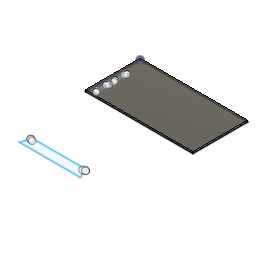
Zaagblad_E (Autodesk Fusion 360 archive; units mm, degrees)
design "Zaagblad_E" references "autodesk generic router xyz"
Autodesk Fusion 360 part; units mm, degrees
sketch "Sketch1" plane through (0, 0, 0) normal (0, 0, 1) x (1, 0, 0)
  line L0 (50.1556, -434.7837) -> (50.1556, -539.8131)
  line L1 (66.9337, -559.4908) -> (52.2058, -544.7629)
  arc A0 (50.1556, -539.8131) -> (52.2058, -544.7629) centre (57.1556, -539.8131) ccw construction
  arc A1 (51.62, -431.2482) -> (50.1556, -434.7837) centre (55.1556, -434.7837) ccw construction
  line L2 (67.2266, -415.6416) -> (51.62, -431.2482) construction
  line L3 (50.1556, -434.7837) -> (50.1556, -539.8131) construction
  line L4 (67.2266, -559.7837) -> (52.2058, -544.7629) construction
  arc A2 (50.1556, -539.8131) -> (52.2058, -544.7629) centre (57.1556, -539.8131) ccw
  arc A3 (51.62, -431.2482) -> (50.1556, -434.7837) centre (55.1556, -434.7837) ccw
  line L5 (66.9337, -415.9345) -> (51.62, -431.2482)
  line L6 (70.1556, -415.6416) -> (70.1556, -559.7837)
  line L7 (67.6408, -559.7837) -> (70.1556, -559.7837)
  arc A4 (66.9337, -559.4908) -> (67.6408, -559.7837) centre (67.6408, -558.7837) ccw
  line L8 (67.6408, -415.6416) -> (70.1556, -415.6416)
  arc A5 (67.6408, -415.6416) -> (66.9337, -415.9345) centre (67.6408, -416.6416) ccw
  line L9 (0, 0) -> (1200, 0)
  line L10 (1200, 0) -> (1200, -610)
  line L11 (1200, -610) -> (0, -610)
  line L12 (0, -610) -> (0, 0)
  line L13 (178.8438, -1361.7664) -> (743.8334, -1361.7664)
  arc A6 (178.8438, -1361.7664) -> (155.3514, -1378.2159) centre (178.8438, -1386.7664) ccw
  line L14 (155.3514, -1378.2159) -> (121.3018, -1471.7664)
  line L15 (121.3018, -1471.7664) -> (801.3753, -1471.7664)
  line L16 (767.3257, -1378.2159) -> (801.3753, -1471.7664)
  arc A7 (767.3257, -1378.2159) -> (743.8334, -1361.7664) centre (743.8334, -1386.7664) ccw
  arc A8 (51.62, -231.2482) -> (50.1556, -234.7837) centre (55.1556, -234.7837) ccw
  line L17 (66.9337, -215.9345) -> (51.62, -231.2482)
  line L18 (67.2266, -359.7837) -> (52.2058, -344.7629) construction
  line L19 (67.6408, -215.6416) -> (70.1556, -215.6416)
  line L20 (67.6408, -359.7837) -> (70.1556, -359.7837)
  line L21 (67.2266, -215.6416) -> (51.62, -231.2482) construction
  arc A9 (66.9337, -359.4908) -> (67.6408, -359.7837) centre (67.6408, -358.7837) ccw
  line L22 (70.1556, -215.6416) -> (70.1556, -359.7837)
  arc A10 (50.1556, -339.8131) -> (52.2058, -344.7629) centre (57.1556, -339.8131) ccw
  arc A11 (67.6408, -215.6416) -> (66.9337, -215.9345) centre (67.6408, -216.6416) ccw
  line L23 (50.1556, -234.7837) -> (50.1556, -339.8131)
  line L24 (50.1556, -234.7837) -> (50.1556, -339.8131) construction
  arc A12 (51.62, -231.2482) -> (50.1556, -234.7837) centre (55.1556, -234.7837) ccw construction
  line L25 (66.9337, -359.4908) -> (52.2058, -344.7629)
  arc A13 (50.1556, -339.8131) -> (52.2058, -344.7629) centre (57.1556, -339.8131) ccw construction
  dimension "d269" = 7
  dimension "d270" = 5
  dimension "d5" = 7
  dimension "d6" = 5
  dimension "d9" = 1
  dimension "d10" = 1
  dimension "d11" = 1200
  dimension "d12" = 610
  dimension "d250" = 25
  dimension "d251" = 25
  dimension "d15" = 7
  dimension "d16" = 5
  dimension "d17" = 7
  dimension "d18" = 5
  dimension "d19" = 1
  dimension "d20" = 1
  constraint tangent L0 A0
  constraint tangent L1 A0
  constraint tangent L0 A1
  constraint tangent A1 L2
  constraint tangent L3 A2
  constraint tangent L4 A2
  constraint tangent L3 A3
  constraint tangent A3 L5
  constraint perpendicular L6 L7
  constraint tangent L1 A4
  constraint tangent L7 A4
  constraint perpendicular L6 L8
  constraint tangent L5 A5
  constraint tangent L8 A5
  constraint horizontal L9
  constraint vertical L10
  constraint horizontal L11
  constraint vertical L12
  constraint coincident L9.start L12.end
  constraint horizontal L13
  constraint tangent L13 A6
  constraint tangent L13 A7
  constraint tangent L23 A13
  constraint tangent L25 A13
  constraint tangent L23 A12
  constraint tangent L21 A12
  constraint tangent A10 L24
  constraint tangent L18 A10
  constraint tangent A8 L24
  constraint tangent A8 L17
  constraint perpendicular L20 L22
  constraint tangent A9 L25
  constraint tangent L20 A9
  constraint perpendicular L19 L22
  constraint tangent L17 A11
  constraint tangent L19 A11
  measures "d269" radius of A0
  measures "d270" radius of A1
  measures "d5" radius of A2
  measures "d6" radius of A3
  measures "d9" radius of A4
  measures "d10" radius of A5
  measures "d11" distance of L9.start L9.end
  measures "d12" distance of L9.start L11.end
  measures "d250" radius of A6
  measures "d251" radius of A7
  measures "d15" radius of A13
  measures "d16" radius of A12
  measures "d17" radius of A10
  measures "d18" radius of A8
  measures "d19" radius of A9
  measures "d20" radius of A11
extrude "Extrude1" add sketch "Sketch1" along normal blind 18 contours L0 L1 A2 A3 L5 L6 L7 A4 L8 A5 | L9 L10 L11 L12 | A8 L17 L19 L20 A9 L22 A10 A11 L23 L25
